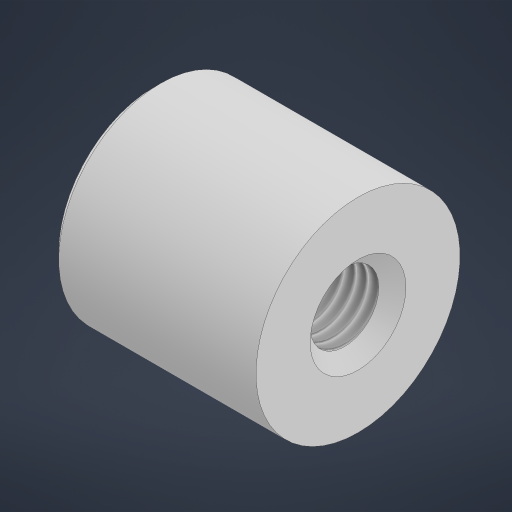
# Autodesk Inventor part: HM1-003X
Saved by Autodesk Inventor 2024.1 (Build 281209000, 209)
## iProperties
Created: 2023-12-03
Part Number: HM1-003X
Material: Generic
Document SubType Name: Modeling
Designer: fablabadmin
Density: 1 g/cm^3
Appearance: Default
Description: Face Insert
Author: fablabadmin
Autodesk Inventor part; units mm, degrees
ref_plane "YZ Plane" through (0, 0, 0) normal (1, 0, 0) x (0, 1, 0)
ref_plane "XZ Plane" through (0, 0, 0) normal (0, 1, 0) x (-1, 0, 0)
ref_plane "XY Plane" through (0, 0, 0) normal (0, 0, 1) x (1, 0, 0)
sketch "Sketch1" plane through (0, 0, 0) normal (0, 0, 1) x (1, 0, 0)
  line L0 (-36, 0) -> (6, 0) projected
  line L1 (0, -3) -> (0, 18) construction
  line L2 (0, 0) -> (0, 15)
  line L3 (0, 15) -> (-30, 15)
  line L4 (-30, 15) -> (-30, 0)
  dimension "d0" = 30
  dimension "d1" = 30
  constraints: 6 end point, 2 point on line, 1 horizontal, 1 perpendicular
  measures "d0" diameter of L3 L0
  measures "d1" distance between parallel lines of L1 L4
revolve "Revolution1" add sketch "Sketch1" angle 360 about axis through (-10, 0, 0) along (1, 0, 0)
sketch "Sketch2" plane through (0, 0, 0) normal (1, 0, 0) x (0, 0, -1)
  circle A0 centre (0, 0) radius 15 projected
  constraints: 1 coincident
hole "Hole1" at (0, 0, 0) direction (-1, 0, 0) diameter 10.106 depth 15 tip angle 118 countersink diameter 14.1 countersink angle 90 thread size "M12x1.75" class "6H" standard "ISO Metric profile"
chamfer "Chamfer1" distance 1 angle 45 1 edges at (-30, -15, 0)
body "Solid1"
